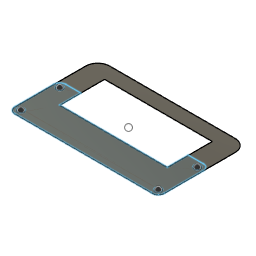
2023_05_23_AppleFootToMultiPurposeHolder v4 (Autodesk Fusion 360 design; units mm, degrees)
Autodesk Fusion 360 part; units mm, degrees
sketch "Imac Flat Holder" plane through (0, 0, 0) normal (0, 0, 1) x (1, 0, 0)
  line L0 (0, 0) -> (55, 0) construction
  line L1 (0, 0) -> (-55, 0) construction
  circle A0 centre (-57.5, 0.0002) radius 2.5
  circle A1 centre (57.5, 0) radius 2.5
  circle A2 centre (57.4995, -32.6078) radius 2.5
  circle A3 centre (-57.5002, -32.4998) radius 2.5
  circle A4 centre (57.5, 0) radius 5
  circle A5 centre (57.4995, -32.6078) radius 5
  circle A6 centre (-57.5002, -32.4998) radius 5
  circle A7 centre (-57.5, 0.0002) radius 5
  line L2 (-57.5434, 5) -> (57.5, 5)
  line L3 (62.4995, -0.069) -> (62.4995, -32.6078)
  line L4 (58.5328, -37.4998) -> (-57.5002, -37.4998)
  line L5 (-62.5, -32.4529) -> (-62.5, 0.0002)
  line L6 (45, -12.5) -> (-45, -12.5)
  line L7 (-45, -12.5) -> (-45, 12.5)
  line L8 (-45, 12.5) -> (45, 12.5)
  line L9 (45, 12.5) -> (45, -12.5)
  line L10 (45, -12.5) -> (-45, 12.5) construction
  line L11 (-45, -12.5) -> (45, 12.5) construction
  line L12 (-57.5, 0.0002) -> (-57.5002, -32.4998)
  line L13 (57.5, 0) -> (57.4995, -32.6078)
  line L14 (-57.5, -2.4998) -> (-57.5002, -29.9998)
  dimension "d1" = 55
  dimension "d2" = 55
  dimension "d8" = 10
  dimension "d12" = 90
  dimension "d13" = 25
  dimension "d16" = 5
  dimension "d17" = 32.5
  dimension "d18" = 27.5
  constraint coincident L0.start L1.start
  constraint horizontal L0
  constraint parallel L0 L1
  constraint coincident L1.end A0
  constraint coincident L0.end A1
  constraint concentric A1 A4
  constraint concentric A2 A5
  constraint concentric A3 A6
  constraint concentric A0 A7
  constraint coincident A7 L2.start
  constraint coincident A4 L2.end
  constraint tangent A4 L2
  constraint horizontal L2
  constraint coincident A4 L3.start
  constraint coincident A5 L3.end
  constraint tangent A5 L3
  constraint perpendicular L2 L3
  constraint coincident A5 L4.start
  constraint coincident A6 L4.end
  constraint tangent A6 L4
  constraint perpendicular L3 L4
  constraint coincident A6 L5.start
  constraint coincident A7 L5.end
  constraint tangent A7 L5
  constraint perpendicular L4 L5
  constraint horizontal L6
  constraint perpendicular L6 L7
  constraint parallel L6 L8
  constraint parallel L7 L9
  constraint coincident L10 L0.start
  constraint coincident L11 L0.start
  constraint equal A1 A2
  constraint equal A1 A3
  constraint equal A0 A1
  constraint equal A4 A5
  constraint equal A4 A6
  constraint equal A4 A7
  constraint coincident A0.centre A7.centre
  constraint coincident A3.centre A6.centre
  constraint coincident A1.centre A4.centre
  constraint coincident A2.centre A5.centre
  constraint coincident A0 L14.start
  constraint coincident L12 L14.start
  constraint coincident A3 L14.end
  constraint coincident L12 L14.end
  measures "d1" distance of L0.start L0.end
  measures "d2" distance of L0.start L1.end
  measures "d8" diameter of A4
  measures "d12" distance of L7.end L8.end
  measures "d13" distance of L6.end L7.end
  measures "d16" diameter of A1
  measures "d17" vertical distance of A0.centre A3.centre
  measures "d18" vertical distance of L14.start L14.end
extrude "Extrude1" add sketch "Imac Flat Holder" along normal blind 0.2 contours A4 | A4 A5 A6 A7 L2 L4 L6 L7 L9 L12 L13 L14 | A4 A5 L3 L13 | A5 L4 | A5 L4 | A7 | A6 | A6 A7 L5 L12 L14 makes body 1
sketch "Imac flat holes measure" plane through (0, 0, 0.2) normal (0, 0, 1) x (-1, 0, 0)
  circle A0 centre (57.5002, 32.4998) radius 2.5
  circle A1 centre (-57.5, 0) radius 2.5
  circle A2 centre (57.5, -0.0002) radius 2.5
  circle A3 centre (-57.4995, 32.6078) radius 2.5
  arc A4 (-56.4662, 37.4998) -> (-62.4995, 32.6078) centre (-57.4995, 32.6078) ccw
  line L0 (-62.4995, 32.6078) -> (-62.4995, 0.069)
  arc A5 (-62.4995, 0.069) -> (-57.5, -5) centre (-57.5, 0) ccw
  line L1 (-57.5, -5) -> (-45, -5)
  line L2 (-45, -5) -> (-45, 12.5)
  line L3 (-45, 12.5) -> (45, 12.5)
  line L4 (45, 12.5) -> (45, -5)
  line L5 (45, -5) -> (57.4566, -5)
  arc A6 (57.4566, -5) -> (62.5, -0.0002) centre (57.5, -0.0002) ccw
  line L6 (62.5, -0.0002) -> (62.5, 32.4529)
  arc A7 (62.5, 32.4529) -> (57.5002, 37.4998) centre (57.5002, 32.4998) ccw
  line L7 (57.5002, 37.4998) -> (-56.4662, 37.4998)
  arc A8 (-62.4995, 0.069) -> (-57.5, -5) centre (-57.5, 0) ccw
  circle A9 centre (57.5, -0.0002) radius 2.5
  arc A10 (-56.4662, 37.4998) -> (-62.4995, 32.6078) centre (-57.4995, 32.6078) ccw
  line L8 (45, -5) -> (57.4566, -5)
  circle A11 centre (-57.5, 0) radius 2.5
  arc A12 (57.4566, -5) -> (62.5, -0.0002) centre (57.5, -0.0002) ccw
  circle A13 centre (-57.4995, 32.6078) radius 2.5
  circle A14 centre (57.5002, 32.4998) radius 2.5
  line L9 (45, 12.5) -> (45, -5)
  line L10 (62.5, -0.0002) -> (62.5, 32.4529)
  arc A15 (62.5, 32.4529) -> (57.5002, 37.4998) centre (57.5002, 32.4998) ccw
  line L11 (-62.4995, 32.6078) -> (-62.4995, 0.069)
  line L12 (-57.5, -5) -> (-45, -5)
  line L13 (-45, 12.5) -> (45, 12.5)
  line L14 (57.5002, 37.4998) -> (-56.4662, 37.4998)
  line L15 (-45, -5) -> (-45, 12.5)
sketch "Sketch3" plane through (0, 0, 0.2) normal (0, 0, 1) x (1, 0, 0)
sketch "Sketch4" plane through (0, 0, 0) normal (1, 0, 0) x (0, 1, 0)
sketch "Sketch5" plane through (0, 0, 0.2) normal (0, 0, 1) x (-1, 0, 0)
  line L0 (45, -5) -> (-45, -5)
  line L1 (-45, -5) -> (-45, -25)
  line L2 (-45, -25) -> (45, -25)
  line L3 (45, -25) -> (45, -5)
  line L4 (57.5002, 37.4998) -> (-56.4662, 37.4998)
  arc A0 (-56.4662, 37.4998) -> (-62.4995, 32.6078) centre (-57.4995, 32.6078) ccw
  line L5 (-62.4995, 32.6078) -> (-62.4995, 0.069)
  arc A1 (-62.4995, 0.069) -> (-57.5, -5) centre (-57.5, 0) ccw
  line L6 (-57.5, -5) -> (-45, -5)
  line L7 (-45, -5) -> (-45, 12.5)
  line L8 (-45, 12.5) -> (45, 12.5)
  line L9 (45, 12.5) -> (45, -5)
  line L10 (45, -5) -> (57.4566, -5)
  arc A2 (57.4566, -5) -> (62.5, -0.0002) centre (57.5, -0.0002) ccw
  line L11 (62.5, -0.0002) -> (62.5, 32.4529)
  arc A3 (62.5, 32.4529) -> (57.5002, 37.4998) centre (57.5002, 32.4998) ccw
  line L12 (62.5, -0.0002) -> (-62.4995, -0.0002)
  line L13 (-62.4995, -0.0002) -> (-62.4995, -26.7523)
  line L14 (-52.4995, -36.7523) -> (52.5, -36.7523)
  line L15 (62.5, -26.7523) -> (62.5, -0.0002)
  arc A4 (52.5, -36.7523) -> (62.5, -26.7523) centre (52.5, -26.7523) ccw
  arc A5 (-62.4995, -26.7523) -> (-52.4995, -36.7523) centre (-52.4995, -26.7523) ccw
  dimension "d19" = 10
  constraint horizontal L0
  constraint vertical L1
  constraint horizontal L2
  constraint vertical L3
  constraint horizontal L12
  constraint vertical L13
  constraint horizontal L14
  constraint vertical L15
  constraint tangent L15 A4
  constraint tangent L14 A4
  constraint tangent L14 A5
  constraint tangent L13 A5
  constraint equal A4 A5
  measures "d19" radius of A4
copy_body "CopyPasteBodies1" bodies 1 makes body 2
move_body "Move1" bodies 2 to x (1, 0, 0) y (0, 1, 0) z (0, 0, 1) at (0, 0, 0)
extrude "Extrude2" add sketch "Sketch5" against normal blind 0.2 contours L1 L2 L3 A1 L6 L10 A2 L13 L14 L15 A4 A5 bodies 2
sketch "Sketch6" plane through (0, 0, 0) normal (0, 0, 1) x (1, 0, 0)
  line L0 (148.5, 105) -> (-148.5, 105)
  line L1 (-148.5, 105) -> (-148.5, -105)
  line L2 (-148.5, -105) -> (148.5, -105)
  line L3 (148.5, -105) -> (148.5, 105)
  line L4 (148.5, 105) -> (-148.5, -105) construction
  line L5 (-148.5, 105) -> (148.5, -105) construction
  dimension "d25" = 297
  dimension "d26" = 210
  constraint horizontal L0
  constraint perpendicular L0 L1
  constraint parallel L0 L2
  constraint parallel L1 L3
  constraint coincident L4 origin
  constraint coincident L5 origin
  measures "d25" distance of L1.end L2.end
  measures "d26" distance of L0.end L1.end
sketch "Sketch7" plane through (0, 0, 0.2) normal (0, 0, 1) x (-1, 0, 0)
  line L0 (62.5, -26.7523) -> (62.5, 32.4529)
  arc A0 (62.5, 32.4529) -> (57.5002, 37.4998) centre (57.5002, 32.4998) ccw
  line L1 (57.5002, 37.4998) -> (-56.4662, 37.4998)
  arc A1 (-56.4662, 37.4998) -> (-62.4995, 32.6078) centre (-57.4995, 32.6078) ccw
  line L2 (-62.4995, 32.6078) -> (-62.4995, 0.069)
  arc A2 (-62.4995, 0.069) -> (-62.4995, -0.069) centre (-57.5, 0) ccw
  line L3 (-62.4995, -0.069) -> (-62.4995, -26.7523)
  arc A3 (-62.4995, -26.7523) -> (-52.4995, -36.7523) centre (-52.4995, -26.7523) ccw
  line L4 (-52.4995, -36.7523) -> (52.5, -36.7523)
  arc A4 (52.5, -36.7523) -> (62.5, -26.7523) centre (52.5, -26.7523) ccw
  circle A5 centre (57.5002, 32.4998) radius 2.5
  circle A6 centre (-57.5, 0) radius 2.5
  circle A7 centre (57.5, -0.0002) radius 2.5
  circle A8 centre (-57.4995, 32.6078) radius 2.5
  line L5 (45, 12.5) -> (45, -25)
  line L6 (45, -25) -> (-45, -25)
  line L7 (-45, -25) -> (-45, 12.5)
  line L8 (-45, 12.5) -> (45, 12.5)
sketch "Imac flat holes measure A4" plane through (0, 0, 0.2) normal (0, 0, 1) x (-1, 0, 0)
  line L0 (62.5, -26.7523) -> (62.5, 32.4529)
  arc A0 (62.5, 32.4529) -> (57.5002, 37.4998) centre (57.5002, 32.4998) ccw
  line L1 (57.5002, 37.4998) -> (-56.4662, 37.4998)
  arc A1 (-56.4662, 37.4998) -> (-62.4995, 32.6078) centre (-57.4995, 32.6078) ccw
  line L2 (-62.4995, 32.6078) -> (-62.4995, 0.069)
  arc A2 (-62.4995, 0.069) -> (-62.4995, -0.069) centre (-57.5, 0) ccw
  line L3 (-62.4995, -0.069) -> (-62.4995, -26.7523)
  arc A3 (-62.4995, -26.7523) -> (-52.4995, -36.7523) centre (-52.4995, -26.7523) ccw
  line L4 (-52.4995, -36.7523) -> (52.5, -36.7523)
  arc A4 (52.5, -36.7523) -> (62.5, -26.7523) centre (52.5, -26.7523) ccw
  circle A5 centre (57.5002, 32.4998) radius 2.5
  circle A6 centre (-57.5, 0) radius 2.5
  circle A7 centre (57.5, -0.0002) radius 2.5
  circle A8 centre (-57.4995, 32.6078) radius 2.5
  line L5 (45, 12.5) -> (45, -25)
  line L6 (45, -25) -> (-45, -25)
  line L7 (-45, -25) -> (-45, 12.5)
  line L8 (-45, 12.5) -> (45, 12.5)
  line L9 (57.5002, 37.4998) -> (-56.4662, 37.4998)
  line L10 (-62.4995, -0.069) -> (-62.4995, -26.7523)
  line L11 (62.5, -26.7523) -> (62.5, 32.4529)
  line L12 (-62.4995, 32.6078) -> (-62.4995, 0.069)
  arc A9 (52.5, -36.7523) -> (62.5, -26.7523) centre (52.5, -26.7523) ccw
  line L13 (-52.4995, -36.7523) -> (52.5, -36.7523)
  line L14 (-45, 12.5) -> (45, 12.5)
  line L15 (45, -25) -> (-45, -25)
  arc A10 (62.5, 32.4529) -> (57.5002, 37.4998) centre (57.5002, 32.4998) ccw
  line L16 (-45, -25) -> (-45, 12.5)
  line L17 (45, 12.5) -> (45, -25)
  circle A11 centre (-57.4995, 32.6078) radius 2.5
  circle A12 centre (57.5, -0.0002) radius 2.5
  arc A13 (-62.4995, -26.7523) -> (-52.4995, -36.7523) centre (-52.4995, -26.7523) ccw
  circle A14 centre (57.5002, 32.4998) radius 2.5
  arc A15 (-56.4662, 37.4998) -> (-62.4995, 32.6078) centre (-57.4995, 32.6078) ccw
  arc A16 (-62.4995, 0.069) -> (-62.4995, -0.069) centre (-57.5, 0) ccw
  circle A17 centre (-57.5, 0) radius 2.5
  line L18 (-148.5, 105) -> (-148.5, -105)
  line L19 (-148.5, -105) -> (148.5, -105)
  line L20 (148.5, -105) -> (148.5, 105)
  line L21 (148.5, 105) -> (-148.5, 105)
  dimension "d27" = 297
  dimension "d28" = 210
  constraint horizontal L21
  constraint perpendicular L18 L21
  constraint parallel L19 L21
  constraint parallel L18 L20
  measures "d27" distance of L19.end L18.end
  measures "d28" distance of L18.start L18.end
hidden bodies 1
equation "d1 = ( 110 / 2 ) * 1 mm"
equation "d2 = ( 110 / 2 ) * 1 mm"
equation "d17 = 27.5 mm + ( 2 * 2.5 ) * 1 mm"
